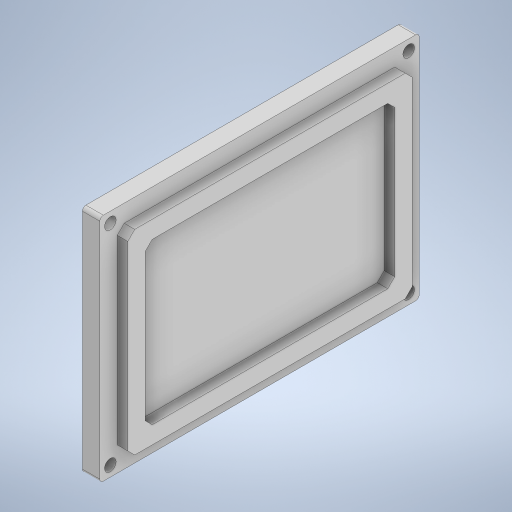
# Autodesk Inventor part: couverclePCB
Saved by Autodesk Inventor 2024 (Build 280153000, 153)
## iProperties
Created: 2023-07-18
Part Number: couverclePCB
Material: Generic
Document SubType Name: Modeling
Designer: pablo
Density: 1 g/cm^3
Appearance: Default
Author: pablo
Autodesk Inventor part; units mm, degrees
ref_plane "YZ Plane" through (0, 0, 0) normal (1, 0, 0) x (0, 1, 0)
ref_plane "XZ Plane" through (0, 0, 0) normal (0, 1, 0) x (-1, 0, 0)
ref_plane "XY Plane" through (0, 0, 0) normal (0, 0, 1) x (1, 0, 0)
sketch "Sketch1" plane through (0, 0, 0) normal (1, 0, 0) x (0, 1, 0)
  line L0 (0, 0) -> (66, 0)
  line L1 (66, 0) -> (66, 91.5)
  line L2 (66, 91.5) -> (0, 91.5)
  line L3 (0, 91.5) -> (0, 0)
  dimension "d0" = 91.5
  dimension "d1" = 66
  constraints: 8 end point, 2 parallel, 1 horizontal, 1 perpendicular
  measures "d0" distance between parallel lines of L0 L2
  measures "d1" distance between parallel lines of L1 L3
extrude "Extrusion1" add sketch "Sketch1" along normal blind 5
fillet "Fillet1" radius 1 4 edges at (2.5, 0, 91.5) (2.5, 0, 0) (2.5, 66, 0) (2.5, 66, 91.5)
sketch "Sketch2" plane through (5, 0, 0) normal (1, 0, 0) x (0, 0, -1)
  line L0 (-86.5, 5) -> (-5, 5)
  line L1 (-5, 5) -> (-5, 61)
  line L2 (-5, 61) -> (-86.5, 61)
  line L3 (-86.5, 61) -> (-86.5, 5)
  line L4 (-90.5, 0) -> (-1, 0) projected
  line L5 (0, 1) -> (0, 65) projected
  line L6 (-1, 66) -> (-90.5, 66) projected
  line L7 (-91.5, 65) -> (-91.5, 1) projected
  point P0 (0, 0)
  dimension "d5" = 5
  dimension "d6" = 5
  dimension "d7" = 5
  dimension "d8" = 5
  constraints: 8 end point, 2 parallel, 1 horizontal, 1 perpendicular
  measures "d5" distance between parallel lines of L4 L0
  measures "d6" distance between parallel lines of L5 L1
  measures "d7" distance between parallel lines of L6 L2
  measures "d8" distance between parallel lines of L7 L3
extrude "Extrusion2" add sketch "Sketch2" along normal blind 3
chamfer "Chamfer1" distance 2 angle 45 4 edges at (6.5, 61, 86.5) (6.5, 5, 86.5) (6.5, 5, 5) (6.5, 61, 5)
sketch "Sketch3" plane through (8, 0, 0) normal (1, 0, 0) x (0, 0, -1)
  line L0 (-81.5, 56) -> (-10, 56)
  line L1 (-10, 56) -> (-10, 10)
  line L2 (-10, 10) -> (-81.5, 10)
  line L3 (-81.5, 10) -> (-81.5, 56)
  line L4 (-5, 7) -> (-5, 59) projected
  line L5 (-7, 61) -> (-84.5, 61) projected
  line L6 (-86.5, 59) -> (-86.5, 7) projected
  line L7 (-84.5, 5) -> (-7, 5) projected
  point P0 (0, 0)
  dimension "d14" = 5
  dimension "d15" = 5
  dimension "d17" = 5
  dimension "d18" = 5
  constraints: 8 end point, 2 parallel, 1 horizontal, 1 perpendicular
  measures "d14" distance between parallel lines of L4 L1
  measures "d15" distance between parallel lines of L5 L0
  measures "d17" distance between parallel lines of L6 L3
  measures "d18" distance between parallel lines of L7 L2
extrude "Extrusion3" cut sketch "Sketch3" against normal blind 3
chamfer "Chamfer2" distance 2 angle 45 4 edges at (6.5, 56, 81.5) (6.5, 56, 10) (6.5, 10, 81.5) (6.5, 10, 10)
sketch "Sketch4" plane through (0, 0, 0) normal (-1, 0, 0) x (0, 0, 1)
  line L0 (3, 3) -> (88.5, 3)
  line L1 (88.5, 3) -> (88.5, 63)
  line L2 (88.5, 63) -> (3, 63)
  line L3 (3, 63) -> (3, 3)
  line L4 (90.5, 0) -> (1, 0) projected
  line L5 (91.5, 65) -> (91.5, 1) projected
  line L6 (1, 66) -> (90.5, 66) projected
  line L7 (0, 1) -> (0, 65) projected
  point P0 (0, 0)
  dimension "d24" = 3
  dimension "d25" = 3
  dimension "d26" = 3
  dimension "d27" = 3
  constraints: 8 end point, 4 coincident, 2 parallel, 1 horizontal, 1 perpendicular
  measures "d24" distance between parallel lines of L4 L0
  measures "d25" distance between parallel lines of L5 L1
  measures "d26" distance between parallel lines of L6 L2
  measures "d27" distance between parallel lines of L7 L3
hole "Hole1" at (0, 63, 88.5) at (0, 3, 88.5) at (0, 3, 3) at (0, 63, 3) direction (1, 0, 0) diameter 3.3 end through all
body "Solid1"
